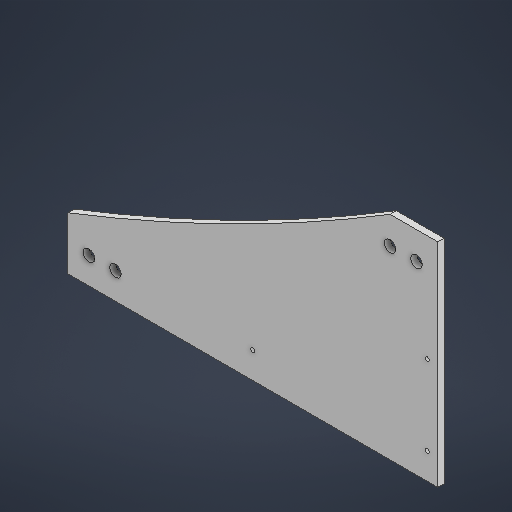
# Autodesk Inventor part: Laser Print For Left Frame with support
Saved by Autodesk Inventor 2026.2 (Build 302298010, 298A)
## iProperties
Created: 2026-04-16
Part Number: Laser Print For Left Frame with support
Material: Generic
Document SubType Name: Sheet Metal
Designer: yassi
Density: 1 g/cm^3
Sheet Metal Rule: Default_mm
Appearance: Default
Author: yassi
Autodesk Inventor part; units mm, degrees
ref_plane "YZ Plane" through (0, 0, 0) normal (1, 0, 0) x (0, 1, 0)
ref_plane "XZ Plane" through (0, 0, 0) normal (0, 1, 0) x (-1, 0, 0)
ref_plane "XY Plane" through (0, 0, 0) normal (0, 0, 1) x (1, 0, 0)
sketch "Sketch1" plane through (0, 0, 0) normal (0, 0, 1) x (1, 0, 0)
  line L0 (0, 0) -> (700, 0)
  line L1 (0, 0) -> (0, 100)
  circle A0 centre (40, 50) radius 10.95
  circle A1 centre (90, 50) radius 10.95
  circle A2 centre (609.6152, 350) radius 10.95
  circle A3 centre (659.6152, 350) radius 10.95
  line L2 (700, 0) -> (700, 402.1837)
  line L3 (700, 402.1837) -> (609.6152, 402.1837)
  arc A4 (0, 100) -> (609.6152, 402.1837) centre (-1371.2256, 3632.2653) ccw
  circle A5 centre (350, 50) radius 3.95
  circle A6 centre (680, 50) radius 3.95
  circle A7 centre (680, 200) radius 3.95
  dimension "d0" = 700
  dimension "d1" = 100
  dimension "d3" = 21.9
  dimension "d5" = 21.9
  dimension "d9" = 21.9
  dimension "d10" = 21.9
  dimension "d14" = 7.9
  dimension "d17" = 7.9
  dimension "d18" = 7.9
  measures "d0" distance of L0.start L0.end
  measures "d1" distance of L0.start L1.end
  measures "d3" diameter of A0
  measures "d5" diameter of A1
  measures "d9" diameter of A2
  measures "d10" diameter of A3
  measures "d14" diameter of A5
  measures "d17" diameter of A6
  measures "d18" diameter of A7
extrude "Plate1" add sketch "Sketch1" along normal blind 12
equation "\"d19\" = Thickness"
equation "\"BendRadius\" = Thickness"
equation "\"BendReliefWidth\" = Thickness"
equation "\"BendReliefDepth\" = 0.5 * Thickness"
equation "\"CornerReliefSize\" = 4 * Thickness"
equation "\"MinimumRemnant\" = 2 * Thickness"
equation "\"TransitionRadius\" = BendRadius"
equation "\"JacobiRadiusSize\" = BendRadius"
equation "\"GapSize\" = Thickness"
equation "\"Thickness\" = 12"
body "Solid1"
